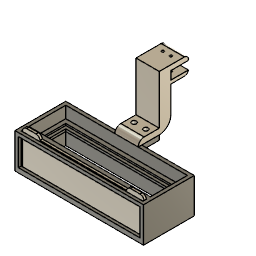
LDR V5 (Autodesk Fusion 360 design; units mm, degrees)
part number: 2025-11-05-08-18-20-954
part number: 2025-11-05-08-36-55-216
part number: 2025-11-05-08-46-39-685
part number: 2025-11-05-08-52-52-138
Autodesk Fusion 360 part; units mm, degrees
note: some values were not read from the file. Set by a fixed rule: which face or edge a step refers to.
sketch "Sketch1" plane through (0, 0, 0) normal (0, 0, 1) x (1, 0, 0)
  line L0 (0, 0) -> (100, 0)
  line L1 (100, 0) -> (100, 31.5)
  line L2 (100, 31.5) -> (0, 31.5)
  line L3 (0, 31.5) -> (0, 0)
  line L4 (-2, -2) -> (102, -2)
  line L5 (102, -2) -> (102, 33.5)
  line L6 (102, 33.5) -> (-2, 33.5)
  line L7 (-2, 33.5) -> (-2, -2)
  line L8 (-5, -5) -> (105, -5)
  line L9 (105, -5) -> (105, 36.5)
  line L10 (105, 36.5) -> (-5, 36.5)
  line L11 (-5, 36.5) -> (-5, -5)
  dimension "d1" = 100
  dimension "d2" = 31.5
  dimension "d3" = 2
  dimension "d4" = 3
  constraint horizontal L0
  constraint vertical L1
  constraint horizontal L2
  constraint vertical L3
  constraint coincident L0.start L3.end
  measures "d1" distance of L0.start L0.end
  measures "d2" distance of L0.start L2.end
extrude "Extrude1" add sketch "Sketch1" along normal blind 30 contours L8 L9 L10 L11 makes body 1
ref_plane "WorkPlane1" through (0, 0, 15) normal (0, 0, 1) x (1, 0, 0)
sketch "Sketch2" plane through (0, 0, 15) normal (0, 0, 1) x (1, 0, 0)
  line L0 (0, 31.5) -> (0, 0)
  line L1 (100, 31.5) -> (0, 31.5)
  line L2 (0, 0) -> (100, 0)
  line L3 (100, 0) -> (100, 31.5)
  line L4 (-2, -2) -> (102, -2)
  line L5 (102, -2) -> (102, 33.5)
  line L6 (102, 33.5) -> (-2, 33.5)
  line L7 (-2, 33.5) -> (-2, -2)
  line L8 (0, 0) -> (-2, 0)
  line L9 (100, 0) -> (102, 0)
  line L10 (102, -2) -> (102, -5)
  line L11 (102, -5) -> (-2, -5)
  line L12 (-2, -5) -> (-2, 0)
  line L13 (-2, 0) -> (102, 0)
  line L14 (102, 0) -> (102, -5)
  dimension "d8" = 2
  constraint coincident L0.end L2.start
  constraint coincident L7 L8.end
  constraint perpendicular L7 L8
  constraint coincident L2.end L3.start
  constraint coincident L5 L9.end
  constraint perpendicular L5 L9
  constraint perpendicular L4 L10
  constraint horizontal L11
  constraint vertical L12
  constraint horizontal L13
  constraint vertical L14
extrude "Extrude2" add sketch "Sketch2" along normal mid plane 2 contours L0 L1 L3 L5 L6 L7 L8 L9 L13 | L2 L4 L5 L7 L8 L9 L12 L13 L14 bodies 1
extrude "Extrude3" cut sketch "Sketch2" along normal mid plane 40 contours L2 L4 L5 L7 L8 L9 L12 L13 L14 | L4 L10 L11 L12 L14 bodies 1
copy_body "Body->Comp2" bodies 1 removing the originals makes body 2 in component "Main"
move_body "Move1" bodies 2 to x (1, 0, 0) y (0, 1, 0) z (0, 0, 1) at (5, 5, 0) in component "Main"
sketch "Sketch1 (2)" plane through (3, 0, 0) normal (1, 0, 0) x (0, 1, 0) in component "Main"
  line L0 (0, 0) -> (38.5, 0)
  line L1 (38.5, 0) -> (38.5, 14)
  line L2 (38.5, 14) -> (5, 14)
  line L3 (5, 14) -> (5, 16)
  line L4 (5, 16) -> (38.5, 16)
  line L5 (38.5, 16) -> (38.5, 30)
  line L6 (38.5, 30) -> (0, 30)
  line L7 (0, 30) -> (0, 0)
  line L8 (5, 16) -> (5, 30) construction
  line L9 (5, 30) -> (0, 30)
  line L10 (0, 30) -> (0, 27)
  line L11 (0, 27) -> (5, 27)
  line L12 (5, 27) -> (5, 30)
  line L13 (0, 30) -> (1.5, 30) construction
  line L14 (5, 30) -> (3.5, 30) construction
  line L15 (3.5, 30) -> (3.5, 27)
  line L16 (1.5, 30) -> (1.5, 27)
  line L17 (5, 14) -> (5, 0) construction
  line L18 (5, 0) -> (0, 0)
  line L19 (0, 0) -> (0, 2)
  line L20 (0, 2) -> (5, 2)
  line L21 (5, 2) -> (5, 0)
  line L22 (5, 2) -> (3.5, 2) construction
  line L23 (3.5, 2) -> (3.5, 4)
  line L24 (3.5, 4) -> (5, 4)
  line L25 (0, 2) -> (0, 4) construction
  line L26 (0, 4) -> (1.5, 4)
  line L27 (1.5, 4) -> (1.5, 2)
  line L28 (5, 4) -> (5, 2)
  line L29 (3.5, 30) -> (1.5, 30)
  line L30 (1.5, 30) -> (1.5, 2)
  line L31 (1.5, 2) -> (3.5, 2)
  line L32 (3.5, 2) -> (3.5, 30)
  dimension "d16" = 1.5
  dimension "d17" = 2
  dimension "d18" = 2
  dimension "d19" = 1.5
  dimension "d20" = 2
  dimension "d21" = 1.5
  dimension "d22" = 3
  dimension "d23" = 1.5
  constraint coincident L3.end L4.start
  constraint coincident L6 L8.end
  constraint perpendicular L6 L8
  constraint horizontal L9
  constraint vertical L10
  constraint horizontal L11
  constraint vertical L12
  constraint coincident L7 L10.end
  constraint coincident L6.end L7.start
  constraint coincident L9 L13.end
  constraint coincident L9 L14.end
  constraint coincident L11 L15.end
  constraint perpendicular L11 L15
  constraint coincident L11 L16.end
  constraint perpendicular L11 L16
  constraint coincident L2.end L3.start
  constraint coincident L0 L17.end
  constraint perpendicular L0 L17
  constraint horizontal L18
  constraint vertical L19
  constraint horizontal L20
  constraint vertical L21
  constraint coincident L7 L19.end
  constraint perpendicular L17 L22
  constraint perpendicular L22 L23
  constraint coincident L17 L24.end
  constraint perpendicular L17 L24
  constraint coincident L7 L25.end
  constraint perpendicular L25 L26
  constraint coincident L20 L27.end
  constraint perpendicular L20 L27
  constraint horizontal L29
  constraint vertical L30
  constraint horizontal L31
  constraint vertical L32
  measures "d16" distance of L20.end L22.end
  measures "d17" distance of L18 L20
  measures "d18" distance of L20 L26
  measures "d19" distance of L25 L27
  measures "d20" distance of L22 L24
  measures "d21" distance of L10 L16
  measures "d22" distance of L11 L13
  measures "d23" distance of L8 L15
sketch "Sketch2 (2)" plane through (107, 0, 0) normal (-1, 0, 0) x (0, -1, 0) in component "Main"
  line L0 (-5, 14) -> (-38.5, 14)
  line L1 (-38.5, 14) -> (-38.5, 0)
  line L2 (-38.5, 0) -> (0, 0)
  line L3 (0, 0) -> (0, 30)
  line L4 (0, 30) -> (-38.5, 30)
  line L5 (-38.5, 30) -> (-38.5, 16)
  line L6 (-38.5, 16) -> (-5, 16)
  line L7 (-5, 16) -> (-5, 14)
  line L8 (-1.5, 30) -> (-1.5, 27)
  line L9 (0, 27) -> (-5, 27)
  line L10 (0, 30) -> (0, 27)
  line L11 (-3.5, 30) -> (-3.5, 27)
  line L12 (-5, 16) -> (-5, 30)
  line L13 (-5, 27) -> (-5, 30)
  line L14 (-5, 30) -> (0, 30)
  line L15 (-1.5, 4) -> (-1.5, 2)
  line L16 (0, 4) -> (-1.5, 4)
  line L17 (0, 2) -> (-5, 2)
  line L18 (0, 0) -> (0, 2)
  line L19 (-5, 0) -> (0, 0)
  line L20 (-3.5, 4) -> (-5, 4)
  line L21 (-3.5, 2) -> (-3.5, 4)
  line L22 (-5, 14) -> (-5, 0)
  line L23 (-1.5, 30) -> (-3.5, 30)
  line L24 (-3.5, 30) -> (-3.5, 2)
  line L25 (-3.5, 2) -> (-1.5, 2)
  line L26 (-1.5, 2) -> (-1.5, 30)
  constraint horizontal L23
  constraint vertical L24
  constraint horizontal L25
  constraint vertical L26
  constraint coincident L21.start L24.end
  constraint coincident L8.start L23.start
extrude "Extrude1'" add sketch "Sketch1 (2)" along normal blind 104 contours L0 L7 L18 L19 L20 L21 L31 bodies 2 in component "Main"
extrude "Extrude2'" add sketch "Sketch1 (2)" along normal blind 104 contours L7 L20 L26 L27 L30 | L20 L23 L24 L28 L32 bodies 2 in component "Main"
extrude "Extrude3'" add sketch "Sketch1 (2)" along normal blind 104 contours L6 L7 L9 L10 L11 L16 L30 | L6 L9 L11 L12 L15 L32 bodies 2 in component "Main"
extrude "Extrude4" add 2 faces at (105.6667, 5, 14.6667) (4.3333, 5, 15.3333) along direction (0, -1, 0) blind 1.5 on bodies 2 bodies 2 in component "Main"
extrude "Extrude5" add 1 faces at (5, 14.5, 15.3333) along direction (1, 0, 0) blind 1.5 on bodies 2 bodies 2 in component "Main"
extrude "Extrude6" add 1 faces at (105, 25.5, 15.3333) along direction (-1, 0, 0) blind 1.5 on bodies 2 bodies 2 in component "Main"
extrude "Extrude7" add 1 faces at (71.1667, 36.5, 14.6667) along direction (0, -1, 0) blind 1.5 on bodies 2 bodies 2 in component "Main"
extrude "Extrude8" add 1 faces at (71.1667, 37.3333, 16) along direction (0, 0, 1) blind 4 on bodies 2 bodies 2 in component "Main"
sketch "Sketch4" plane through (0, 3.5, 0) normal (0, -1, 0) x (1, 0, 0)
  line L0 (103.5, 14) -> (107, 14)
  line L1 (107, 14) -> (107, 20)
  line L2 (107, 20) -> (103.5, 20)
  line L3 (103.5, 20) -> (103.5, 14)
  line L4 (3, 18.5) -> (107, 18.5)
  line L5 (107, 18.5) -> (107, 16)
  line L6 (107, 16) -> (3, 16)
  line L7 (3, 16) -> (3, 18.5)
  dimension "d40" = 2.5
  constraint horizontal L4
  constraint vertical L5
  constraint horizontal L6
  constraint vertical L7
  constraint coincident L1 L5.end
  measures "d40" distance of L4.start L6.end
extrude "Extrude9" cut sketch "Sketch4" against normal blind 35 contours L3 L4 L6 L7 | L1 L3 L4 L5 L6 bodies 2 in component "Main"
sketch "Sketch5" plane through (0, 0, 30) normal (0, 0, 1) x (-1, 0, 0)
  line L0 (0, 0) -> (-110, 0)
  line L1 (-110, 0) -> (-110, -41.5)
  line L2 (-110, -41.5) -> (0, -41.5)
  line L3 (0, -41.5) -> (0, 0)
  line L4 (-107, -1.5) -> (-3, -1.5)
  line L5 (-3, -1.5) -> (-3, -3.5)
  line L6 (-3, -3.5) -> (-107, -3.5)
  line L7 (-107, -3.5) -> (-107, -1.5)
  line L8 (-107, -5) -> (-3, -5)
  line L9 (-3, -5) -> (-3, -38.5)
  line L10 (-3, -38.5) -> (-107, -38.5)
  line L11 (-107, -38.5) -> (-107, -5)
extrude "Extrude1''" add sketch "Sketch5" against normal blind 28 separate body contours L4 L5 L6 L7 makes body 3 in component "Slide"
sketch "Sketch6" plane through (0, 0, 30) normal (0, 0, 1) x (-1, 0, 0)
  line L0 (-107, -3.5) -> (-3, -3.5)
  line L1 (-3, -3.5) -> (-3, -1.5)
  line L2 (-3, -1.5) -> (-107, -1.5)
  line L3 (-107, -1.5) -> (-107, -3.5)
  line L4 (-3, -3.5) -> (-18, -3.5)
  line L5 (-18, -3.5) -> (-18, -1.5)
  line L6 (-18, -1.5) -> (-3, -1.5)
  line L7 (-3, -1.5) -> (-3, -3.5)
  line L8 (-107, -3.5) -> (-92, -3.5)
  line L9 (-92, -3.5) -> (-92, -1.5)
  line L10 (-92, -1.5) -> (-107, -1.5)
  line L11 (-107, -1.5) -> (-107, -3.5)
  dimension "d45" = 15
  dimension "d46" = 15
  constraint horizontal L4
  constraint vertical L5
  constraint horizontal L6
  constraint vertical L7
  constraint coincident L0.end L1.start
  constraint horizontal L8
  constraint vertical L9
  constraint horizontal L10
  constraint vertical L11
  constraint coincident L0.start L3.end
  measures "d45" distance of L0.end L4.end
  measures "d46" distance of L0.start L8.end
extrude "Extrude2''" add sketch "Sketch6" along normal blind 3 contours L0 L2 L3 L8 L9 L10 L11 | L0 L1 L2 L4 L5 L6 L7 bodies 3 in component "Slide"
fillet "Fillet1" radius 3.5 4 edges at (18, 2.5, 33) (3, 2.5, 33) (92, 2.5, 33) (107, 2.5, 33) on bodies 3 in component "Slide"
sketch "Sketch7" plane through (0, 0, 30) normal (0, 0, 1) x (-1, 0, 0)
  line L0 (0, 0) -> (-110, 0)
  line L1 (-110, 0) -> (-110, -41.5)
  line L2 (-110, -41.5) -> (0, -41.5)
  line L3 (0, -41.5) -> (0, 0)
  line L4 (-107, -1.5) -> (-3, -1.5)
  line L5 (-3, -1.5) -> (-3, -3.5)
  line L6 (-3, -3.5) -> (-107, -3.5)
  line L7 (-107, -3.5) -> (-107, -1.5)
  line L8 (-107, -5) -> (-3, -5)
  line L9 (-3, -5) -> (-3, -38.5)
  line L10 (-3, -38.5) -> (-107, -38.5)
  line L11 (-107, -38.5) -> (-107, -5)
  line L12 (-110, -41.5) -> (-55, -41.5) construction
  line L13 (-55, -41.5) -> (-65, -41.5)
  line L14 (-65, -41.5) -> (-45, -41.5)
  line L15 (-45, -41.5) -> (-45, -56.5)
  line L16 (-45, -56.5) -> (-65, -56.5)
  line L17 (-65, -56.5) -> (-65, -41.5)
  circle A0 centre (-60, -50) radius 2
  circle A1 centre (-50, -50) radius 2
  dimension "d51" = 15
  constraint coincident L1.end L2.start
  constraint midpoint L2 L12.end
  constraint coincident L12 L13.end
  constraint horizontal L14
  constraint vertical L15
  constraint horizontal L16
  constraint vertical L17
  measures "d51" distance of L13.end L16.end
extrude "Extrude10" add sketch "Sketch7" against normal blind 4 contours L2 L13 L14 L15 L16 L17 bodies 2 in component "Main"
sketch "Sketch8" plane through (0, 0, 30) normal (0, 0, 1) x (-1, 0, 0)
  circle A0 centre (-60, -50) radius 2
  circle A1 centre (-50, -50) radius 2
  line L0 (0, 0) -> (-110, 0)
  line L1 (-110, 0) -> (-110, -41.5)
  line L2 (-110, -41.5) -> (-65, -41.5)
  line L3 (-65, -41.5) -> (-65, -56.5)
  line L4 (-65, -56.5) -> (-45, -56.5)
  line L5 (-45, -56.5) -> (-45, -41.5)
  line L6 (-45, -41.5) -> (0, -41.5)
  line L7 (0, -41.5) -> (0, 0)
  line L8 (-107, -1.5) -> (-3, -1.5)
  line L9 (-3, -1.5) -> (-3, -3.5)
  line L10 (-3, -3.5) -> (-107, -3.5)
  line L11 (-107, -3.5) -> (-107, -1.5)
  line L12 (-107, -5) -> (-3, -5)
  line L13 (-3, -5) -> (-3, -38.5)
  line L14 (-3, -38.5) -> (-107, -38.5)
  line L15 (-107, -38.5) -> (-107, -5)
  circle A2 centre (-60, -50) radius 2
  circle A3 centre (-50, -50) radius 2
  line L16 (-65, -38.5) -> (-45, -38.5)
  line L17 (-45, -38.5) -> (-45, -56.5)
  line L18 (-45, -56.5) -> (-65, -56.5)
  line L19 (-65, -56.5) -> (-65, -38.5)
  constraint horizontal L16
  constraint vertical L17
  constraint horizontal L18
  constraint vertical L19
  constraint coincident L4.end L5.start
  constraint coincident L14 L16.start
extrude "Extrude1'''" add sketch "Sketch8" along normal blind 5 separate body contours L3 L4 L5 L14 L16 L17 L18 L19 makes body 4 in component "Connector"
fillet "Fillet1'" radius 5 1 edges at (55, 38.5, 35) on bodies 4 in component "Connector"
extrude "Extrude2'''" add 1 faces at (58.3333, 56.5, 33.3333) along direction (0, 1, 0) blind 10 on bodies 4 bodies 4 in component "Connector"
sketch "Sketch9" plane through (0, 0, 35) normal (0, 0, 1) x (-1, 0, 0)
  line L0 (-45, -43.5) -> (-65, -43.5)
  line L1 (-65, -43.5) -> (-65, -66.5)
  line L2 (-65, -66.5) -> (-45, -66.5)
  line L3 (-45, -66.5) -> (-45, -43.5)
  circle A0 centre (-60, -50) radius 2
  circle A1 centre (-50, -50) radius 2
  line L4 (-45, -66.5) -> (-65, -66.5)
  line L5 (-65, -66.5) -> (-65, -56.5)
  line L6 (-65, -56.5) -> (-45, -56.5)
  line L7 (-45, -56.5) -> (-45, -66.5)
  dimension "d60" = 20
  dimension "d61" = 10
  constraint horizontal L4
  constraint vertical L5
  constraint horizontal L6
  constraint vertical L7
  constraint coincident L2.end L3.start
  measures "d60" distance of L2.end L1.end
  measures "d61" distance of L2.end L6.end
extrude "Extrude3''" add sketch "Sketch9" along normal blind 42 contours L1 L2 L3 L4 L5 L6 L7 bodies 4 in component "Connector"
fillet "Fillet2" radius 10 1 edges at (55, 66.5, 30) on bodies 4 in component "Connector"
sketch "Sketch10" plane through (0, 66.5, 0) normal (0, 1, 0) x (-1, 0, 0)
  line L0 (-65, 40) -> (-45, 40)
  line L1 (-45, 40) -> (-45, 77)
  line L2 (-45, 77) -> (-65, 77)
  line L3 (-65, 77) -> (-65, 40)
  line L4 (-45, 77) -> (-65, 77)
  line L5 (-65, 77) -> (-65, 74)
  line L6 (-65, 74) -> (-45, 74)
  line L7 (-45, 74) -> (-45, 77)
  line L8 (-45, 74) -> (-65, 74)
  line L9 (-65, 74) -> (-65, 65.65)
  line L10 (-65, 65.65) -> (-45, 65.65)
  line L11 (-45, 65.65) -> (-45, 74)
  line L12 (-45, 65.65) -> (-65, 65.65)
  line L13 (-65, 65.65) -> (-65, 62.65)
  line L14 (-65, 62.65) -> (-45, 62.65)
  line L15 (-45, 62.65) -> (-45, 65.65)
  dimension "d66" = 3
  dimension "d67" = 8.35
  dimension "d68" = 3
  constraint horizontal L4
  constraint vertical L5
  constraint horizontal L6
  constraint vertical L7
  constraint coincident L1.end L2.start
  constraint horizontal L8
  constraint vertical L9
  constraint horizontal L10
  constraint vertical L11
  constraint horizontal L12
  constraint vertical L13
  constraint horizontal L14
  constraint vertical L15
  measures "d66" distance of L1.end L6.end
  measures "d67" distance of L6.end L10.end
  measures "d68" distance of L10.end L14.end
extrude "Extrude4'" add sketch "Sketch10" along normal blind 15 contours L1 L3 L10 L12 L13 L14 L15 | L1 L2 L3 L4 L5 L6 L7 L8 bodies 4 in component "Connector"
fillet "Fillet3" radius 3.5 2 edges at (55, 81.5, 77) (55, 81.5, 62.65) on bodies 4 in component "Connector"
extrude "Extrude11" cut sketch "Sketch1 (2)" against normal blind 0.04 contours L11 L20 L23 L27 L30 L31 L32 | L6 L9 L11 L15 L16 L29 L30 L32 bodies 2 in component "Main"
extrude "Extrude12" cut sketch "Sketch2 (2)" against normal blind 0.04 contours L9 L15 L17 L21 L24 L25 L26 | L4 L8 L9 L11 L14 L23 L24 L26 bodies 2 in component "Main"
extrude "Extrude13" cut 8 faces at (37.6667, 3.5, 29) (2.9733, 3.5, 15.6667) (107.0267, 3.5, 15.6667) (37.6667, 3.5, 2.6667) (5.3333, 3.5, 15.3333) (5.3333, 3.5, 19.5) (105.8333, 3.5, 19.5) (104.6667, 3.5, 15.3333) along direction (0, 1, 0) blind 0.04 on bodies 2 bodies 2 in component "Main"
extrude "Extrude14" cut 1 faces at (37.6667, 1.5, 29) along direction (0, -1, 0) blind 0.04 on bodies 2 bodies 2 in component "Main"
extrude "Extrude15" add 1 faces at (37.6667, 5, 28) along direction (0, 1, 0) blind 2 on bodies 2 bodies 2 in component "Main"
extrude "Extrude16" add 1 faces at (36.6667, 0, 1.3333) along direction (0, -1, 0) blind 2 on bodies 2 bodies 2 in component "Main"
extrude "Extrude17" cut 1 faces at (37.6667, 1.46, 29) along direction (0, -1, 0) blind 1 on bodies 2 bodies 2 in component "Main"
extrude "Extrude5'" add 1 faces at (58.3333, 76.5, 74) along direction (0, 0, -1) blind 3 on bodies 4 bodies 4 in component "Connector"
extrude "Extrude6'" cut 1 faces at (58.3333, 76.5, 71) along direction (0, 0, 1) blind 3 on bodies 4 bodies 4 in component "Connector"
extrude "Extrude7'" add 1 faces at (58.3333, 76.5, 74) along direction (0, 0, -1) blind 2 on bodies 4 bodies 4 in component "Connector"
extrude "Extrude8'" cut 1 faces at (58.3333, 76.5, 72) along direction (0, 0, 1) blind 0.7 on bodies 4 bodies 4 in component "Connector"
sketch "Sketch11" plane through (0, 0, 77) normal (0, 0, 1) x (-1, 0, 0)
  line L0 (-65, -78.0359) -> (-45, -78.0359)
  line L1 (-45, -78.0359) -> (-45, -56.5)
  line L2 (-45, -56.5) -> (-65, -56.5)
  line L3 (-65, -56.5) -> (-65, -78.0359)
  line L4 (-65, -73) -> (-45, -73) construction
  line L5 (-55, -73) -> (-57.5, -73) construction
  line L6 (-55, -73) -> (-52.5, -73) construction
  circle A0 centre (-58.5, -73) radius 1
  circle A1 centre (-51.5, -73) radius 1
  dimension "d95" = 2.5
  dimension "d96" = 2.5
  dimension "d97" = 2
  dimension "d98" = 2
  constraint coincident L3 L4.start
  constraint coincident L1 L4.end
  constraint perpendicular L1 L4
  constraint midpoint L4 L5.start
  constraint parallel L4 L5
  constraint parallel L4 L6
  constraint coincident L5.end A0
  constraint coincident L6.end A1
  measures "d95" distance of L5.start L5.end
  measures "d96" distance of L5.start L6.end
  measures "d97" diameter of A0
  measures "d98" diameter of A1
extrude "Extrude9'" cut sketch "Sketch11" against normal blind 19 contours A0 | A1 bodies 4 in component "Connector"
component "Main" placed x (1, 0, 0) y (0, 1, 0) z (0, 0, 1) at (0, 0, 0)
component "Slide" placed x (1, 0, 0) y (0, 1, 0) z (0, 0, 1) at (0, 0, 0)
component "Connector" placed x (1, 0, 0) y (0, 1, 0) z (0, 0, 1) at (0, 0, 0)
